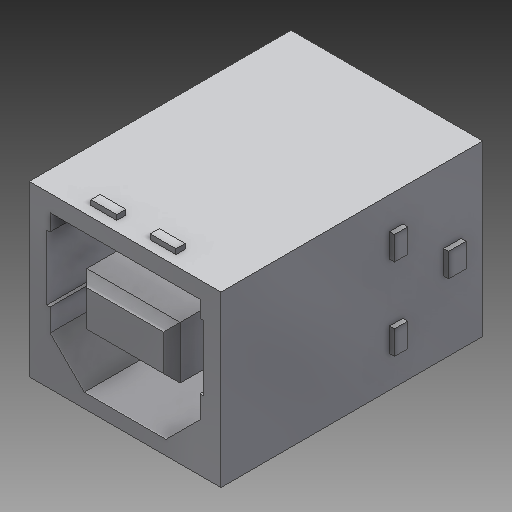
# Autodesk Inventor part: USB Series B Receptacle Housing
Saved by Autodesk Inventor 2017 SP1 (Build 210196100, 196)
## iProperties
Created: 2012-05-07
Material: Nylon, molybdenum disulphide
Document SubType Name: Modeling
Designer: sdarley
Density: 1 g/cm^3
Project: USB Series B Receptacle
Description: USB Series B Receptacle Housing
Appearance: Gładki - Biały
Author: sdarley
Title: USB Series B Receptacle Housing
Revision Number: 1
Autodesk Inventor part; units mm, degrees
ref_plane "YZ Plane" through (0, 0, 0) normal (1, 0, 0) x (0, 1, 0)
ref_plane "XZ Plane" through (0, 0, 0) normal (0, 1, 0) x (-1, 0, 0)
ref_plane "XY Plane" through (0, 0, 0) normal (0, 0, 1) x (1, 0, 0)
sketch "Sketch1" plane through (0, 0, 0) normal (0, 0, 1) x (1, 0, 0)
  line L0 (-5.75, -5.075) -> (5.75, -5.075)
  line L1 (5.75, -5.075) -> (5.75, 5.075)
  line L2 (5.75, 5.075) -> (-5.75, 5.075)
  line L3 (-5.75, 5.075) -> (-5.75, -5.075)
  line L4 (-5.75, -5.075) -> (5.75, 5.075) construction
  line L5 (5.75, -5.075) -> (-5.75, 5.075) construction
  point P0 (0, 0)
  dimension "d0" = 11.5
  dimension "d1" = 10.15
  constraints: 12 end point, 2 midpoint, 2 parallel, 1 horizontal, 1 perpendicular
  measures "d0" distance of L2.end L1.end
  measures "d1" distance of L1.end L0.end
ref_plane "Work Plane1" through (3.5021, -0.15, 11.0247) normal (-0.0829156, 0, -0.9965566) x (0, 1, 0)
extrude "Extrusion1" add sketch "Sketch1" along normal blind 7.2
sketch "Sketch2" plane through (0, 0, 7.2) normal (0, 0, 1) x (1, 0, 0)
  line L0 (-5.75, -5.075) -> (5.75, -5.075) projected
  line L1 (5.75, -5.075) -> (5.75, 5.075) projected
  line L2 (5.75, 5.075) -> (-5.75, 5.075) projected
  line L3 (-5.75, 5.075) -> (-5.75, -5.075) projected
  line L4 (-4.5, 4.075) -> (4.5, 4.075)
  line L5 (-4.5, -2.175) -> (-2.45, -4.225)
  line L6 (2.45, -4.225) -> (4.5, -2.175)
  line L7 (-2.45, -4.225) -> (2.45, -4.225)
  line L8 (-4.5, 3.075) -> (-4.7, 3.075)
  line L9 (-4.5, -0.825) -> (-4.7, -0.825)
  line L10 (4.5, 3.075) -> (4.7, 3.075)
  line L11 (4.5, -0.825) -> (4.7, -0.825)
  line L12 (4.7, -0.825) -> (4.7, 3.075)
  line L13 (-4.7, -0.825) -> (-4.7, 3.075)
  line L14 (-4.5, 4.075) -> (-4.5, 3.075)
  line L15 (-4.5, -0.825) -> (-4.5, -2.175)
  line L16 (4.5, 4.075) -> (4.5, 3.075)
  line L17 (4.5, -0.825) -> (4.5, -2.175)
  line L18 (-2.8, 1.775) -> (2.8, 1.775)
  line L19 (2.8, 1.775) -> (2.8, -1.375)
  line L20 (2.8, -1.375) -> (-2.8, -1.375)
  line L21 (-2.8, -1.375) -> (-2.8, 1.775)
  point P0 (0, 0)
  point P1 (4.5, -2.175)
  point P2 (0, 4.075)
  point P3 (0, 1.775)
  dimension "d6" = 3.9
  dimension "d8" = 1
  dimension "d9" = 9.4
  dimension "d10" = 0.2
  dimension "d11" = 3.15
  dimension "d12" = 5.6
  dimension "d13" = 2.3
  constraints: 36 end point, 9 perpendicular, 6 vertical, 3 horizontal, 3 horizontal alignment, 3 parallel, 3 vertical alignment, 2 midpoint, 2 point on line, 2 other
  measures "d6" distance between parallel lines of L10 L11
  measures "d8" distance between parallel lines of L4 L10
  measures "d9" distance between parallel lines of L13 L12
  measures "d10" distance between parallel lines of L17 L12
  measures "d11" distance of L18.end L19.end
  measures "d12" distance of L18.start L18.end
  measures "d13" distance between parallel lines of L4 L18
ref_plane "Work Plane2" through (3.5021, -0.15, 11.0247) normal (-0.0829156, 0, -0.9965566) x (0, 1, 0)
ref_plane "Work Plane3" through (-5.75, -5.075, 15.7) normal (0, 0, -1) x (0, 1, 0)
extrude "Extrusion2" add sketch "Sketch2" along normal up to surface (8.5 mm away)
chamfer "Chamfer1" distance 0.5 angle 45 4 edges at (0, -1.375, 15.7) (-2.8, 0.2, 15.7) (0, 1.775, 15.7) (2.8, 0.2, 15.7)
sketch "Sketch3" plane through (0, 0, 7.2) normal (0, 0, 1) x (1, 0, 0)
  line L0 (-2.8, 1.775) -> (2.8, 1.775) projected
  line L1 (2.8, -1.375) -> (-2.8, -1.375) projected
  line L2 (-1.925, 2.925) -> (-0.575, 2.925)
  line L3 (-0.575, 2.925) -> (-0.575, 1.475)
  line L4 (-0.575, 1.475) -> (-1.925, 1.475)
  line L5 (-1.925, 1.475) -> (-1.925, 2.925)
  line L6 (0.575, 2.925) -> (1.925, 2.925)
  line L7 (1.925, 2.925) -> (1.925, 1.475)
  line L8 (1.925, 1.475) -> (0.575, 1.475)
  line L9 (0.575, 1.475) -> (0.575, 2.925)
  line L10 (-1.925, -1.075) -> (-0.575, -1.075)
  line L11 (-0.575, -1.075) -> (-0.575, -2.525)
  line L12 (-0.575, -2.525) -> (-1.925, -2.525)
  line L13 (-1.925, -2.525) -> (-1.925, -1.075)
  line L14 (0.575, -1.075) -> (1.925, -1.075)
  line L15 (1.925, -1.075) -> (1.925, -2.525)
  line L16 (1.925, -2.525) -> (0.575, -2.525)
  line L17 (0.575, -2.525) -> (0.575, -1.075)
  point P0 (0, 0)
  point P1 (0, 1.775)
  point P2 (-1.25, 2.925)
  point P3 (1.25, 2.925)
  dimension "d17" = 1.35
  dimension "d19" = 1.45
  dimension "d20" = 1.15
  dimension "d21" = 1.15
  dimension "d22" = 2.5
  dimension "d23" = 1.25
  constraints: 32 end point, 8 parallel, 6 equal length, 4 horizontal, 4 perpendicular, 3 midpoint, 2 horizontal alignment, 2 vertical alignment
  measures "d17" distance of L2.start L2.end
  measures "d19" distance of L4.end L2.start
  measures "d20" distance between parallel lines of L0 L2
  measures "d21" distance between parallel lines of L1 L12
  measures "d22" distance of point (1.25, 2.925) point (-1.25, 2.925)
  measures "d23" horizontal distance of point (0, 1.775) point (-1.25, 2.925)
extrude "Extrusion3" cut sketch "Sketch3" against normal blind 6.5 and the other way blind 5.8
sketch "Sketch4" plane through (-5.75, 5.075, 0) normal (0, 1, 0) x (1, 0, 0)
  line L0 (11.5, -15.7) -> (0, -15.7) projected
  line L1 (3.1, -15.1) -> (3.1, -14.55)
  line L2 (3.1, -14.55) -> (4.65, -14.55)
  line L3 (4.65, -14.55) -> (4.65, -15.1)
  line L4 (6.65, -15.1) -> (6.65, -14.55)
  line L5 (6.65, -14.55) -> (8.2, -14.55)
  line L6 (8.2, -14.55) -> (8.2, -15.1)
  line L7 (3.1, -15.1) -> (4.65, -15.1)
  line L8 (6.65, -15.1) -> (8.2, -15.1)
  dimension "d28" = 0.6
  constraints: 16 end point, 4 vertical, 2 horizontal, 2 perpendicular, 1 horizontal alignment, 4 other
  measures "d28" distance between parallel lines of L7 L0
ref_plane "Work Plane4" through (-6.05, 5.375, -0.3) normal (0, 1, 0) x (0, 0, 1)
extrude "Extrusion4" add sketch "Sketch4" along normal up to surface (0.3 mm away)
sketch "Sketch5" plane through (-5.75, -5.075, 0) normal (-1, 0, 0) x (0, 0, 1)
  line L0 (1, 5.75) -> (2.35, 5.75)
  line L1 (2.45, 4.4) -> (2.45, 5.65)
  line L2 (0.9, 4.4) -> (0.9, 5.65)
  line L3 (1, 4.3) -> (2.35, 4.3)
  line L4 (4.8, 6.8) -> (6.15, 6.8)
  line L5 (6.25, 8.15) -> (6.25, 6.9)
  line L6 (4.8, 8.25) -> (6.15, 8.25)
  line L7 (4.7, 6.9) -> (4.7, 8.15)
  line L8 (4.8, 3.35) -> (6.15, 3.35)
  line L9 (4.7, 3.25) -> (4.7, 2)
  line L10 (6.25, 3.25) -> (6.25, 2)
  line L11 (6.15, 1.9) -> (4.8, 1.9)
  line L12 (4.8, 8.24) -> (5.6, 8.24)
  line L13 (5.6, 8.24) -> (5.6, 6.81)
  line L14 (5.6, 6.81) -> (4.8, 6.81)
  line L15 (4.8, 6.81) -> (4.8, 8.24)
  line L16 (4.8, 3.34) -> (5.6, 3.34)
  line L17 (5.6, 3.34) -> (5.6, 1.91)
  line L18 (5.6, 1.91) -> (4.8, 1.91)
  line L19 (4.8, 1.91) -> (4.8, 3.34)
  line L20 (1.3, 5.74) -> (2.35, 5.74)
  line L21 (2.35, 5.74) -> (2.35, 4.31)
  line L22 (2.35, 4.31) -> (1.3, 4.31)
  line L23 (1.3, 4.31) -> (1.3, 5.74)
  dimension "d31" = 0.65
  dimension "d33" = 0.01
  dimension "d34" = 0.01
  dimension "d35" = 0.65
  dimension "d36" = 0.01
  dimension "d37" = 0.01
  dimension "d38" = 0.4
  dimension "d39" = 0.01
  dimension "d40" = 0.01
  constraints: 48 end point, 9 horizontal, 6 parallel, 6 vertical, 3 perpendicular, 3 vertical alignment, 24 other
  measures "d31" distance between parallel lines of L5 L13
  measures "d33" distance between parallel lines of L6 L12
  measures "d34" distance between parallel lines of L4 L14
  measures "d35" distance between parallel lines of L10 L17
  measures "d36" distance between parallel lines of L16 L8
  measures "d37" distance between parallel lines of L11 L18
  measures "d38" distance between parallel lines of L2 L23
  measures "d39" distance between parallel lines of L0 L20
  measures "d40" distance between parallel lines of L3 L22
ref_plane "Work Plane5" through (-6.05, -5.375, -0.3) normal (-1, 0, 0) x (0, 0, 1)
extrude "Extrusion5" add sketch "Sketch5" along normal up to surface (0.3 mm away)
mirror "Mirror1" about plane through (0, 0, 0) normal (1, 0, 0) of "Extrusion5"
equation "\"d21\" = d20"
equation "\"d23\" = 0.5 * d22"
equation "\"d34\" = d33"
equation "\"d35\" = d31"
equation "\"d36\" = d33"
equation "\"d37\" = d36"
equation "\"d39\" = d33"
equation "\"d40\" = d39"
body "Solid1"
